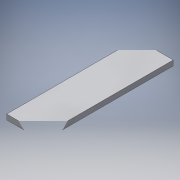
# Autodesk Inventor part: soprte bateria parte 2
Saved by Autodesk Inventor 2016 (Build 200138000, 138)
## iProperties
Created: 2017-03-11
Part Number: soprte bateria parte 2
Material: Generic
Document SubType Name: Modeling
Designer: jorge
Density: 1 g/cm^3
Appearance: White
Author: jorge
Autodesk Inventor part; units mm, degrees
ref_plane "YZ Plane" through (0, 0, 0) normal (1, 0, 0) x (0, 1, 0)
ref_plane "XZ Plane" through (0, 0, 0) normal (0, 1, 0) x (-1, 0, 0)
ref_plane "XY Plane" through (0, 0, 0) normal (0, 0, 1) x (1, 0, 0)
sketch "Sketch1" plane through (0, 0, 0) normal (0, 0, 1) x (1, 0, 0)
  arc A0 (31, 0) -> (31, 20) centre (31, 10) ccw projected
  line L0 (10, 20) -> (31, 20) projected
  arc A1 (10, 20) -> (10, 0) centre (10, 10) ccw projected
  line L1 (31, 0) -> (10, 0) projected
  arc A2 (10, 23) -> (10, -3) centre (10, 10) ccw
  line L2 (10, 23) -> (31, 23)
  arc A3 (31, -3) -> (31, 23) centre (31, 10) ccw
  line L3 (31, -3) -> (10, -3)
  line L4 (31, 20) -> (31, 23)
  line L5 (10, 20) -> (10, 23)
  point P0 (0, 0)
  dimension "d0" = 3
  constraints: 8 end point, 4 point on circle, 2 centre point, 1 point on line, 1 vertical, 3 other
  measures "d0" distance between parallel lines of L1 L3
ref_plane "Work Plane1" through (-41.8096, -51.8081, -71) normal (0, 0, -1) x (-0.6474127, 0.7621396, 0)
extrude "Extrusion1" add sketch "Sketch1" against normal up to surface (71 mm away) contours L0 L5 L2 L4
sketch "Sketch2" plane through (0, 0, 0) normal (0, 0, 1) x (1, 0, 0)
  line L0 (31, 20) -> (31, 23) projected
  line L1 (31, 23) -> (10, 23) projected
  line L2 (10, 23) -> (10, 20) projected
  line L3 (10, 20) -> (31, 20) projected
  point P0 (0, 0)
ref_plane "Work Plane2" through (40.6247, -21.3797, 4) normal (0, 0, 1) x (0.7621396, 0.6474127, 0)
extrude "Extrusion2" add sketch "Sketch2" along normal up to surface (4 mm away)
body "Solid1"
